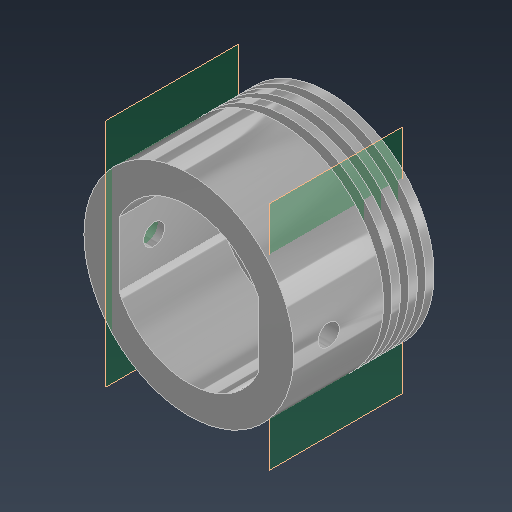
# Autodesk Inventor part: P003-Corps_piston
Saved by Autodesk Inventor 2021.3 (Build 253353000, 353)
## iProperties
Company: HES-SO
Created: 2022-03-18
Part Number: P003-Corps_piston
Material: Aluminium
Document SubType Name: Modeling
Designer: Rémi & Elise
Density: 2.7 g/cm^3
Appearance: Aluminum - Dark
Mass: 21.5358 g
Surface Area: 56.8938 cm^2
Volume: 7.9762 cm^3
Author: Rémi & Elise
Title: Corps piston
Autodesk Inventor part; units mm, degrees
ref_plane "XZ Plane" through (0, 0, 0) normal (0, 1, 0) x (-1, 0, 0)
ref_plane "XY Plane" through (0, 0, 0) normal (0, 0, 1) x (1, 0, 0)
sketch "Sketch5" plane through (0, 0, 0) normal (0, 0, 1) x (1, 0, 0)
  line L0 (-17.9489, 0) -> (2.9915, 0) construction
  line L1 (0, -4) -> (0, 24) construction
  line L2 (-10.9575, 0) -> (-10.9575, 15)
  line L3 (-10.9575, 15) -> (0, 15)
  line L4 (0, 20) -> (-14.9575, 20)
  line L5 (-14.9575, 20) -> (-14.9575, 18.8)
  line L6 (-14.9575, 18.8) -> (-12.9575, 18.8)
  line L7 (-12.9575, 18.8) -> (-12.9575, 17.6)
  line L8 (-12.9575, 17.6) -> (-14.9575, 17.6)
  line L9 (-14.9575, 17.6) -> (-14.9575, 16.4)
  line L10 (-14.9575, 16.4) -> (-12.9575, 16.4)
  line L11 (-12.9575, 16.4) -> (-12.9575, 15.2)
  line L12 (-12.9575, 15.2) -> (-14.9575, 15.2)
  line L13 (-14.9575, 15.2) -> (-14.9575, 14)
  line L14 (-14.9575, 14) -> (-12.9575, 14)
  line L15 (0, 20) -> (0, 15)
  line L16 (-12.9575, 14) -> (-12.9575, 12.8)
  line L17 (-12.9575, 12.8) -> (-14.9575, 12.8)
  line L18 (-14.9575, 12.8) -> (-14.9575, 0)
  line L19 (-14.9575, 0) -> (-10.9575, 0)
  point P0 (0, 0)
  dimension "d18" = 1.2
  dimension "d35" = 5
  dimension "d38" = 2
  dimension "d39" = 2
  dimension "d42" = 29.9149
  dimension "d49" = 15
  constraints: 36 end point, 11 perpendicular, 10 point on line, 5 parallel, 2 collinear, 2 vertical, 1 horizontal
  measures "d18" distance of L6.end L7.end
  measures "d35" distance of L4.start L3.end
  measures "d38" distance of L16.end L17.end
  measures "d39" distance between parallel lines of L2 L16
  measures "d42" diameter of L5 L1
  measures "d49" distance of L2.start L2.end
revolve "Revolution1" add sketch "Sketch5" angle 360 about axis through (0, -10, 0) along (0, 1, 0)
ref_plane "Work Plane1" through (20, 0, 0) normal (1, 0, 0) x (0, 1, 0)
sketch "Sketch6" plane through (20, 0, 0) normal (1, 0, 0) x (0, 1, 0)
  line L0 (14, -14.9575) -> (14, 14.9575) construction
  line L1 (15.2, -14.9575) -> (15.2, 14.9575) construction
  line L2 (16.4, -12.9575) -> (16.4, 12.9575) construction
  line L3 (16.4, -14.9575) -> (16.4, 14.9575) construction
  line L4 (17.6, -14.9575) -> (17.6, 14.9575) construction
  line L5 (17.6, -12.9575) -> (17.6, 12.9575) construction
  line L6 (18.8, -12.9575) -> (18.8, 12.9575) construction
  line L7 (18.8, -14.9575) -> (18.8, 14.9575) construction
  line L8 (20, -14.9575) -> (20, 14.9575) construction
  line L9 (-4, 0) -> (24, 0) construction
  line L10 (0, -14.9575) -> (0, 14.9575) construction
  point P0 (0, 0)
  point P1 (5, -17.5)
  point P2 (5, 17.5)
  point P3 (5, 0)
  dimension "d41" = 5
  constraints: 1 point on line
  measures "d41" distance from line of point (5, 0) L10
hole "Hole1" at (20, 5, 0) direction (-1, 0, 0) diameter 3 end through all
ref_plane "Work Plane3" through (10.9575, 7.5, 0) normal (-1, 0, 0) x (0, -1, 0)
ref_plane "Work Plane2" through (-14.2908, 5, 0) normal (-1, 0, 0) x (0, -0.4233179, 0.9059812)
sketch "Sketch7" plane through (10.9575, 7.5, 0) normal (-1, 0, 0) x (0, -1, 0)
  spline S0 degree 7 poles (1, 0) (1, -0.1802) (1.0252, -0.3572) (1.0742, -0.5267) (1.1441, -0.6845) (1.2315, -0.8273) (1.3317, -0.953) (1.6813, -1.3027) (1.9706, -1.463) (2.2784, -1.5461) (2.5916, -1.5582) (2.9012, -1.5016) (3.1992, -1.369) (3.5855, -1.0487) (3.7082, -0.9188) (3.8168, -0.7663) (3.9049, -0.5936) (3.9674, -0.4047) (4, -0.2048) (4, 0.2049) (3.9674, 0.4048) (3.9049, 0.5936) (3.8168, 0.7663) (3.7082, 0.9188) (3.5856, 1.0487) (3.3351, 1.2559) (3.2054, 1.3383) (3.0696, 1.4034) (2.9298, 1.4518) (2.7874, 1.4839) (2.6437, 1.5) (2.3563, 1.5) (2.2126, 1.4839) (2.0702, 1.4518) (1.9304, 1.4034) (1.7946, 1.3383) (1.6649, 1.2559) (1.4145, 1.0487) (1.2918, 0.9188) (1.1832, 0.7663) (1.095, 0.5936) (1.0326, 0.4047) (1, 0.2048) (1, 0) knots 0 0 0 0 0 0 0 0 0.114256 0.114256 0.114256 0.114256 0.114256 0.114256 0.371167 0.371167 0.371167 0.371167 0.371167 0.371167 0.500252 0.500252 0.500252 0.500252 0.500252 0.500252 0.629363 0.629363 0.629363 0.629363 0.629363 0.629363 0.750149 0.750149 0.750149 0.750149 0.750149 0.750149 0.870934 0.870934 0.870934 0.870934 0.870934 0.870934 1 1 1 1 1 1 1 1 projected
  line L0 (7.5, 14.9575) -> (7.5, -14.9575) construction
  line L1 (-5.3, 14.9575) -> (-5.3, -14.9575) construction
  line L2 (-7.5, 7.5) -> (7.5, 7.5)
  line L3 (7.5, 7.5) -> (7.5, -7.5)
  line L4 (7.5, -7.5) -> (-7.5, -7.5)
  line L5 (-7.5, -7.5) -> (-7.5, 7.5)
  circle A0 centre (2.5, 0) radius 1.5 construction
  line L6 (-7.5, 10.9575) -> (-7.5, -10.9575) construction
  line L7 (-7.5, 7.5) -> (7.5, -7.5) construction
  line L8 (7.5, 7.5) -> (-7.5, -7.5) construction
  point P0 (7.5, 0)
  point P1 (0, 0)
  dimension "d43" = 3
  constraints: 12 end point, 3 perpendicular, 2 collinear, 2 parallel, 1 horizontal, 1 horizontal alignment, 1 midpoint, 2 other
  measures "d43" diameter of A0
extrude "Extrusion4" add sketch "Sketch7" along normal blind 1
ref_plane "Work Plane4" through (-10.9575, 0, 0) normal (-1, 0, 0) x (0, -1, 0)
sketch "Sketch8" plane through (-10.9575, 0, 0) normal (-1, 0, 0) x (0, -1, 0)
  line L0 (-15, 4.5733) -> (0, 4.5733) projected
  line L1 (-15, -4.5733) -> (-15, 4.5733) projected
  line L2 (0, -4.5733) -> (-15, -4.5733) projected
  line L3 (0, -4.5733) -> (0, 4.5733) projected
  circle A0 centre (-5, 0) radius 1.5 projected
  point P0 (0, 0)
extrude "Extrusion5" add sketch "Sketch8" against normal blind 1
body "Solid3"
